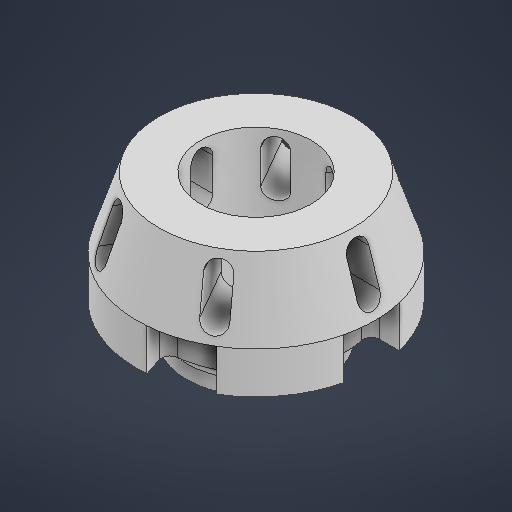
# Autodesk Inventor part: b11
Saved by Autodesk Inventor 2025.4 (Build 294407000, 407)
## iProperties
Created: 2026-05-15
Part Number: b11
Material: Generic
Document SubType Name: Modeling
Designer: VuQuan
Density: 1 g/cm^3
Appearance: Default
Author: VuQuan
Autodesk Inventor part; units mm, degrees
ref_plane "YZ Plane" through (0, 0, 0) normal (1, 0, 0) x (0, 1, 0)
ref_plane "XZ Plane" through (0, 0, 0) normal (0, 1, 0) x (-1, 0, 0)
ref_plane "XY Plane" through (0, 0, 0) normal (0, 0, 1) x (1, 0, 0)
sketch "Sketch1" plane through (0, 0, 0) normal (0, 0, 1) x (1, 0, 0)
  line L0 (0, 0) -> (0, 52.5)
  line L1 (0, 0) -> (-25, 0)
  line L2 (-25, 0) -> (-25, 5)
  line L3 (-25, 5) -> (-32.5, 12.5)
  line L4 (-32.5, 12.5) -> (-43, 12.5)
  line L5 (-43, 12.5) -> (-43, 27.5)
  line L6 (-43, 27.5) -> (-35, 52.5)
  line L7 (-35, 52.5) -> (0, 52.5)
  dimension "d0" = 5
  dimension "d1" = 50
  dimension "d2" = 86
  dimension "d3" = 52.5
  dimension "d4" = 12.5
  dimension "d5" = 45
  dimension "d6" = 70
  dimension "d7" = 15
  constraints: 16 end point, 2 parallel, 2 perpendicular, 1 horizontal, 1 vertical
  measures "d0" distance of L1.end L2.end
  measures "d1" diameter of L2 L0
  measures "d2" diameter of L5 L0
  measures "d3" distance between parallel lines of L7 L1
  measures "d4" distance between parallel lines of L4 L1
  measures "d5" angle of L1 L3
  measures "d6" diameter of L6.end L0
  measures "d7" distance of L4.end L5.end
revolve "Revolution1" add sketch "Sketch1" angle 360 about axis through (0, 0, 0) along (0, 1, 0)
sketch "Sketch2" plane through (0, 52.5, 0) normal (0, 1, 0) x (1, 0, 0)
  circle A0 centre (0, 0) radius 35 projected
  circle A1 centre (0, 0) radius 20
  dimension "d9" = 40
  constraints: 1 centre point, 1 coincident
  measures "d9" diameter of A1
extrude "Extrusion1" cut sketch "Sketch2" against normal through all contours A1
sketch "Sketch3" plane through (0, 0, 0) normal (1, 0, 0) x (0, 1, 0)
  line L0 (46, 0) -> (34, 0) construction
  line L1 (46, 4) -> (34, 4)
  line L2 (34, -4) -> (46, -4)
  arc A0 (46, -4) -> (46, 4) centre (46, 0) ccw
  arc A1 (34, 4) -> (34, -4) centre (34, 0) ccw
  line L3 (12.5, -43) -> (12.5, 43) projected
  point P0 (0, 0)
  point P1 (40, 0)
  dimension "d12" = 12
  dimension "d14" = 8
  dimension "d15" = 21.5
  constraints: 8 end point, 4 point on circle, 4 tangent, 2 centre point, 1 horizontal, 1 midpoint, 1 parallel, 1 point on line
  measures "d12" distance of L0.start L0.end
  measures "d14" distance between parallel lines of L1 L2
  measures "d15" distance from line of L3 L0.end
extrude "Extrusion2" cut sketch "Sketch3" against normal up to surface
pattern_circular "Circular Pattern1" count 6 over 360 about axis through (0, -10, 0) along (0, 1, 0) of "Extrusion2"
sketch "Sketch4" plane through (0, 12.5, 0) normal (0, -1, 0) x (1, 0, 0)
  circle A0 centre (0, 0) radius 32.5 projected
  circle A1 centre (0, 0) radius 43 projected
  line L0 (41.821, 10) -> (34.803, 10)
  arc A2 (34.803, 10) -> (31.8619, 6.4085) centre (34.803, 7) ccw
  line L1 (41.821, -10) -> (34.803, -10)
  arc A3 (31.8619, -6.4085) -> (34.803, -10) centre (34.803, -7) ccw
  line L2 (32.5, 0) -> (43, 0) construction
  circle A4 centre (0, 0) radius 43 projected
  dimension "d21" = 3
  dimension "d22" = 20
  constraints: 10 point on circle, 6 end point, 4 tangent, 3 horizontal, 2 centre point, 1 equal radius, 1 point on line, 1 other
  measures "d21" radius of A2
  measures "d22" distance between parallel lines of L1 L0
extrude "Extrusion3" cut sketch "Sketch4" against normal blind 15 contours A0 A2 L0 A1 L1 A3 picked at (36.4979, 6.9963)
pattern_circular "Circular Pattern2" count 5 over 360 about axis through (0, -10, 0) along (0, 1, 0) of "Extrusion3"
body "Solid1"
